Autodesk Fusion 360 part; units mm, degrees
note: some values were not read from the file. Set by a fixed rule: which face or edge a step refers to.
(part 4 of 4)
sketch "Sketch2 (2)" plane through (0, 0, 5) normal (0, 0, 1) x (-1, 0, 0)
  line L0 (3.02, 3.0627) -> (-2.5, 1.0536)
  line L1 (-2.5, 1.0536) -> (-2.5, -1.0536)
  line L2 (-2.5, -1.0536) -> (3.02, -3.0627)
  line L3 (3.02, -3.0627) -> (3.02, -4.7913)
  line L4 (3.02, -4.7913) -> (-2.5, -6.8004)
  line L5 (-2.5, -6.8004) -> (-2.5, -8.9076)
  line L6 (-2.5, -8.9076) -> (3.02, -10.9167)
  line L7 (3.02, -10.9167) -> (3.02, -12.6453)
  line L8 (3.02, -12.6453) -> (-2.5, -14.6544)
  line L9 (-2.5, -14.6544) -> (-2.5, -16.7615)
  line L10 (-2.5, -16.7615) -> (3.02, -18.7706)
  line L11 (3.02, -18.7706) -> (3.02, -20.4993)
  line L12 (3.02, -20.4993) -> (-2.5, -22.5084)
  line L13 (-2.5, -22.5084) -> (-2.5, -24.6155)
  line L14 (-2.5, -24.6155) -> (3.02, -26.6246)
  line L15 (3.02, -26.6246) -> (3.02, -28.3532)
  line L16 (3.02, -28.3532) -> (-2.5, -30.3624)
  line L17 (-2.5, -30.3624) -> (-2.5, -32.4695)
  line L18 (-2.5, -32.4695) -> (3.02, -34.4786)
  line L19 (3.02, -34.4786) -> (3.02, -36.2072)
  line L20 (3.02, -36.2072) -> (-2.5, -38.2163)
  line L21 (-2.5, -38.2163) -> (-2.5, -40.3235)
  line L22 (-2.5, -40.3235) -> (3.02, -42.3326)
  line L23 (3.02, -42.3326) -> (3.02, -44.0612)
  line L24 (3.02, -44.0612) -> (-2.5, -46.0703)
  line L25 (-2.5, -46.0703) -> (-2.5, -48.1775)
  line L26 (-2.5, -48.1775) -> (3.02, -50.1866)
  line L27 (3.02, -50.1866) -> (3.02, -51.9152)
  line L28 (3.02, -51.9152) -> (-2.5, -53.9243)
  line L29 (-2.5, -53.9243) -> (-2.5, -56.0314)
  line L30 (-2.5, -56.0314) -> (3.02, -58.0406)
  line L31 (3.02, -58.0406) -> (3.02, -59.7692)
  line L32 (3.02, -59.7692) -> (-2.5, -61.7783)
  line L33 (-2.5, -61.7783) -> (-2.5, -63.8854)
  line L34 (-2.5, -63.8854) -> (3.02, -65.8945)
  line L35 (3.02, -65.8945) -> (3.02, -67.6231)
  line L36 (3.02, -67.6231) -> (-2.5, -69.6323)
  line L37 (-2.5, -69.6323) -> (-2.5, -71.7394)
  line L38 (-2.5, -71.7394) -> (3.02, -73.7485)
  line L39 (3.02, -73.7485) -> (3.02, -75.4771)
  line L40 (3.02, -75.4771) -> (-2.5, -77.4862)
  line L41 (-2.5, -77.4862) -> (-2.5, -79.5934)
  line L42 (-2.5, -79.5934) -> (3.02, -81.6025)
  line L43 (3.02, -81.6025) -> (3.02, -83.3311)
  line L44 (3.02, -83.3311) -> (-2.5, -85.3402)
  line L45 (-2.5, -85.3402) -> (-2.5, -87.4474)
  line L46 (-2.5, -87.4474) -> (3.02, -89.4565)
  line L47 (3.02, -89.4565) -> (3.02, -91.1851)
  line L48 (3.02, -91.1851) -> (-2.5, -93.1942)
  line L49 (-2.5, -93.1942) -> (-2.5, -95.3013)
  line L50 (-2.5, -95.3013) -> (3.02, -97.3105)
  line L51 (3.02, -97.3105) -> (3.02, -99.0391)
  line L52 (3.02, -99.0391) -> (-2.5, -101.0482)
  line L53 (-2.5, -101.0482) -> (-2.5, -103.1553)
  line L54 (-2.5, -103.1553) -> (3.02, -105.1644)
  line L55 (3.02, -105.1644) -> (3.02, -106.8931)
  line L56 (3.02, -106.8931) -> (-2.5, -108.9022)
  line L57 (-2.5, -108.9022) -> (-2.5, -111.0093)
  line L58 (-2.5, -111.0093) -> (3.02, -113.0184)
  line L59 (3.02, -113.0184) -> (3.02, -114.747)
  line L60 (3.02, -114.747) -> (-2.5, -116.7562)
  line L61 (-2.5, -116.7562) -> (-2.5, -118.8633)
  line L62 (-2.5, -118.8633) -> (3.02, -120.8724)
  line L63 (3.02, -120.8724) -> (3.02, -122.601)
  line L64 (3.02, -122.601) -> (-2.5, -124.6101)
  line L65 (-2.5, -124.6101) -> (-2.5, -126.7173)
  line L66 (-2.5, -126.7173) -> (3.02, -128.7264)
  line L67 (3.02, -128.7264) -> (3.02, -130.455)
  line L68 (3.02, -130.455) -> (-2.5, -132.4641)
  line L69 (-2.5, -132.4641) -> (-2.5, -134.5713)
  line L70 (-2.5, -134.5713) -> (3.02, -136.5804)
  line L71 (3.02, -136.5804) -> (3.02, -138.309)
  line L72 (3.02, -138.309) -> (-2.5, -140.3181)
  line L73 (-2.5, -140.3181) -> (-2.5, -142.4252)
  line L74 (-2.5, -142.4252) -> (3.02, -144.4344)
  line L75 (3.02, -144.4344) -> (3.02, -146.163)
  line L76 (3.02, -146.163) -> (-2.5, -148.1721)
  line L77 (-2.5, -148.1721) -> (-2.5, -150.2792)
  line L78 (-2.5, -150.2792) -> (3.02, -152.2883)
  line L79 (3.02, -152.2883) -> (3.02, -154.0169)
  line L80 (3.02, -154.0169) -> (-2.5, -156.0261)
  line L81 (-2.5, -156.0261) -> (-2.5, -158.1332)
  line L82 (-2.5, -158.1332) -> (3.02, -160.1423)
  line L83 (3.02, -160.1423) -> (3.02, -161.8709)
  line L84 (3.02, -161.8709) -> (-2.5, -163.88)
  line L85 (-2.5, -163.88) -> (-2.5, -165.9872)
  line L86 (-2.5, -165.9872) -> (3.02, -167.9963)
  line L87 (3.02, -167.9963) -> (3.02, -169.7249)
  line L88 (3.02, -169.7249) -> (-2.5, -171.734)
  line L89 (-2.5, -171.734) -> (-2.5, -173.8412)
  line L90 (-2.5, -173.8412) -> (3.02, -175.8503)
  line L91 (3.02, -175.8503) -> (3.02, -177.5789)
  line L92 (3.02, -177.5789) -> (-2.5, -179.588)
  line L93 (-2.5, -179.588) -> (-2.5, -181.6951)
  line L94 (-2.5, -181.6951) -> (3.02, -183.7043)
  line L95 (3.02, -183.7043) -> (3.02, -184.5686)
  line L96 (3.02, -184.5686) -> (13.02, -184.5686)
  line L97 (13.02, -184.5686) -> (13.02, 18.927)
  line L98 (13.02, 18.927) -> (-76.98, 18.927)
  line L99 (-76.98, 18.927) -> (-76.98, 3.927)
  line L100 (-76.98, 3.927) -> (3.02, 3.927)
  line L101 (3.02, 3.927) -> (3.02, 3.0627)
  line L102 (-31.98, 18.927) -> (-31.98, 3.927) construction
  line L103 (-76.98, 3.927) -> (-31.98, 18.927) construction
  line L104 (13.02, 3.927) -> (-31.98, 18.927) construction
  line L105 (-36.98, 15.177) -> (-26.98, 15.177)
  line L106 (-26.98, 15.177) -> (-26.98, 7.677)
  line L107 (-26.98, 7.677) -> (-36.98, 7.677)
  line L108 (-36.98, 7.677) -> (-36.98, 15.177)
  line L109 (-36.98, 15.177) -> (-26.98, 7.677) construction
  line L110 (-26.98, 15.177) -> (-36.98, 7.677) construction
  line L111 (-14.48, 15.177) -> (-4.48, 15.177)
  line L112 (-4.48, 15.177) -> (-4.48, 7.677)
  line L113 (-4.48, 7.677) -> (-14.48, 7.677)
  line L114 (-14.48, 7.677) -> (-14.48, 15.177)
  line L115 (-14.48, 15.177) -> (-4.48, 7.677) construction
  line L116 (-4.48, 15.177) -> (-14.48, 7.677) construction
  point P0 (-31.98, 11.427)
  point P1 (-54.48, 11.427)
  point P2 (-9.48, 11.427)
  dimension "d8" = 10
  dimension "d9" = 7.5
  dimension "d12" = 10
  dimension "d13" = 7.5
  constraint midpoint L98 L102.start
  constraint coincident L100 L102.end
  constraint perpendicular L100 L102
  constraint coincident L99.end L100.start
  constraint coincident L97 L104.start
  constraint horizontal L105
  constraint perpendicular L105 L106
  constraint parallel L105 L107
  constraint parallel L106 L108
  constraint coincident L109 P0
  constraint coincident L110 P0
  constraint midpoint L102 P0
  constraint midpoint L103 P1
  constraint horizontal L111
  constraint perpendicular L111 L112
  constraint parallel L111 L113
  constraint parallel L112 L114
  constraint coincident L115 P2
  constraint coincident L116 P2
  constraint midpoint L104 P2
  measures "d8" distance of L105.start L105.end
  measures "d9" distance of L105.start L107.end
  measures "d12" distance of L111.start L111.end
  measures "d13" distance of L111.end L112.end
extrude "Extrude3" cut sketch "Sketch2 (2)" against normal blind 10 contours L105 L106 L107 L108 | L111 L112 L113 L114 in component "Rack; Module: 2.50 mm; Num Teeth: 24; Pressure Angle: 20 deg; Backlash: 0.00 mm;"
sketch "Sketch3" plane through (0, -18.927, 0) normal (0, -1, 0) x (1, 0, 0)
  line L0 (76.98, 5) -> (-13.02, 5)
  line L1 (-13.02, 5) -> (-13.02, -5)
  line L2 (-13.02, -5) -> (76.98, -5)
  line L3 (76.98, -5) -> (76.98, 5)
  line L4 (31.98, 5) -> (31.98, -5) construction
  line L5 (-13.02, 5) -> (31.98, -5) construction
  line L6 (76.98, 5) -> (31.98, -5) construction
  circle A0 centre (31.98, 0) radius 1.5
  circle A1 centre (9.48, 0) radius 1.5
  dimension "d16" = 3
  dimension "d17" = 3
  constraint midpoint L0 L4.start
  constraint midpoint L2 L4.end
  constraint coincident L0.end L1.start
  constraint coincident L0.start L3.end
  constraint midpoint L4 A0.centre
  constraint midpoint L5 A1.centre
  measures "d16" diameter of A1
  measures "d17" diameter of A0
extrude "Extrude4" cut sketch "Sketch3" against normal blind 15 contours A0 | A1 in component "Rack; Module: 2.50 mm; Num Teeth: 24; Pressure Angle: 20 deg; Backlash: 0.00 mm;"
extrude "Extrude5" cut 1 faces at (76.98, -8.927, -1.6667) along direction (-1, 0, 0) blind 20 in component "Rack; Module: 2.50 mm; Num Teeth: 24; Pressure Angle: 20 deg; Backlash: 0.00 mm;"
sketch "Sketch4" plane through (0, 184.5686, 0) normal (0, 1, 0) x (-1, 0, 0)
  line L0 (13.02, -5) -> (13.02, 5)
  line L1 (13.02, 5) -> (3.02, 5)
  line L2 (3.02, 5) -> (3.02, -5)
  line L3 (3.02, -5) -> (13.02, -5)
  line L4 (13.02, 5) -> (-13, 5)
  line L5 (-13, 5) -> (-13, -5)
  line L6 (-13, -5) -> (13.02, -5)
  line L7 (13.02, -5) -> (13.02, 5)
  constraint perpendicular L4 L5
  constraint parallel L4 L6
  constraint parallel L5 L7
  constraint perpendicular L0 L4
  constraint coincident L0.end L1.start
extrude "Extrude6" cut sketch "Sketch4" against normal blind 31 in component "Rack; Module: 2.50 mm; Num Teeth: 24; Pressure Angle: 20 deg; Backlash: 0.00 mm;"
component "Rack; Module: 2.50 mm; Num Teeth: 24; Pressure Angle: 20 deg; Backlash: 0.00 mm;" placed x (1, 0, 0) y (0, 1, 0) z (0, 0, 1) at (0, 0, 0)

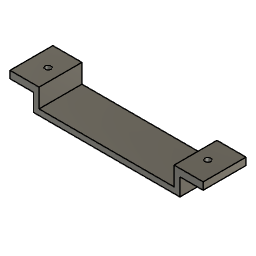
design "bracket"
Autodesk Fusion 360 part; units mm, degrees
sketch "Sketch1" plane through (0, 0, 0) normal (0, 0, 1) x (1, 0, 0)
  line L0 (50.5, -44.75) -> (-50.5, -44.75)
  line L1 (-50.5, -44.75) -> (-50.5, 44.75)
  line L2 (-50.5, 44.75) -> (50.5, 44.75)
  line L3 (50.5, 44.75) -> (50.5, -44.75)
  line L4 (50.5, -44.75) -> (-50.5, 44.75) construction
  line L5 (-50.5, -44.75) -> (50.5, 44.75) construction
  dimension "d1" = 101
  dimension "d2" = 89.5
  constraint horizontal L0
  constraint perpendicular L0 L1
  constraint parallel L0 L2
  constraint parallel L1 L3
  constraint coincident L4 origin
  constraint coincident L5 origin
  measures "d1" distance of L1.end L2.end
  measures "d2" distance of L0.end L1.end
extrude "Extrude1" add sketch "Sketch1" along normal blind 12
shell "Shell1" thickness 4 removed faces 1 at (-16.8333, 14.9167, 12)
extrude "Extrude2" cut 1 faces at (15.5, 40.75, 6.6667) along direction (0, -1, 0) up to surface (85.5 mm away) and the other way up to surface (4 mm away)
sketch "Sketch3" plane through (0, 0, 12) normal (0, 0, 1) x (-1, 0, 0)
  line L0 (46.5, 44.75) -> (46.5, -44.75)
  line L1 (46.5, -44.75) -> (50.5, -44.75)
  line L2 (50.5, -44.75) -> (50.5, 44.75)
  line L3 (50.5, 44.75) -> (46.5, 44.75)
  line L4 (46.5, -44.75) -> (66.5, -44.75)
  line L5 (66.5, -44.75) -> (66.5, 44.75)
  line L6 (66.5, 44.75) -> (46.5, 44.75)
  line L7 (46.5, 44.75) -> (46.5, -44.75)
  line L8 (0, -2.5) -> (0, -20)
  line L9 (-46.5, -44.75) -> (-66.5, -44.75)
  line L10 (-66.5, -44.75) -> (-66.5, 44.75)
  line L11 (-46.5, 44.75) -> (-46.5, -44.75)
  line L12 (-66.5, 44.75) -> (-46.5, 44.75)
  line L13 (0, 0) -> (55, 0) construction
  circle A0 centre (55, 0) radius 2
  circle A1 centre (-55, 0) radius 2
  dimension "d15" = 89.5
  dimension "d16" = 20
  dimension "d21" = 55
  dimension "d22" = 4
  constraint perpendicular L4 L5
  constraint parallel L4 L6
  constraint parallel L5 L7
  constraint perpendicular L2 L4
  constraint coincident L0.end L1.start
  constraint symmetric L0.end L8 L9.start
  constraint symmetric L4.end L8 L9.end
  constraint symmetric L5.end L8 L10.end
  constraint symmetric L0.start L8 L11.start
  constraint coincident L13.start origin
  constraint perpendicular L2 L13
  constraint coincident L13.end A0.centre
  constraint symmetric L8 A0 A1
  measures "d15" distance of L4.end L5.end
  measures "d16" distance of L5.end L0.start
  measures "d21" distance of L13.start L13.end
  measures "d22" diameter of A0
extrude "Extrude4" add sketch "Sketch3" along normal blind 5
move_face "OffsetFaces1" offset -30 1 faces at (54.5, -44.75, 15.3333)
move_face "OffsetFaces2" offset -30 1 faces at (54.5, 44.75, 15.3333)

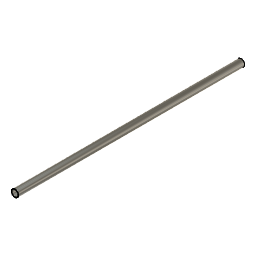
design "axle"
Autodesk Fusion 360 part; units mm, degrees
sketch "Sketch1" plane through (0, 0, 0) normal (0, 1, 0) x (1, 0, 0)
  circle A0 centre (0, 0) radius 4
  circle A1 centre (0, 0) radius 3.5
  dimension "d1" = 8
  dimension "d2" = 7
  constraint coincident A0.centre A1.centre
  measures "d1" diameter of A0
  measures "d2" diameter of A1
extrude "Extrude1" add sketch "Sketch1" along normal mid plane 250

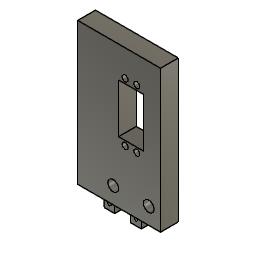
design "servo_side_stand"
Autodesk Fusion 360 part; units mm, degrees
sketch "Sketch1" plane through (0, 0, 0) normal (0, 0, 1) x (1, 0, 0)
  line L0 (45, -7.5) -> (-45, -7.5) construction
  line L1 (-45, -7.5) -> (-45, 7.5) construction
  line L2 (-45, 7.5) -> (45, 7.5) construction
  line L3 (45, 7.5) -> (45, -7.5) construction
  line L4 (45, -7.5) -> (-45, 7.5) construction
  line L5 (-45, -7.5) -> (45, 7.5) construction
  line L6 (0, -7.5) -> (45, 7.5) construction
  line L7 (-45, 7.5) -> (0, -7.5) construction
  line L8 (4.5, -3.25) -> (-4.5, -3.25)
  line L9 (-4.5, -3.25) -> (-4.5, 3.25)
  line L10 (-4.5, 3.25) -> (4.5, 3.25)
  line L11 (4.5, 3.25) -> (4.5, -3.25)
  line L12 (4.5, -3.25) -> (-4.5, 3.25) construction
  line L13 (-4.5, -3.25) -> (4.5, 3.25) construction
  line L14 (-27, -3.25) -> (-18, -3.25)
  line L15 (-18, -3.25) -> (-18, 3.25)
  line L16 (-18, 3.25) -> (-27, 3.25)
  line L17 (-27, 3.25) -> (-27, -3.25)
  line L18 (-27, -3.25) -> (-18, 3.25) construction
  line L19 (-18, -3.25) -> (-27, 3.25) construction
  point P0 (22.5, 0)
  point P1 (-22.5, 0)
  dimension "d1" = 90
  dimension "d2" = 15
  dimension "d3" = 9
  dimension "d4" = 9
  dimension "d7" = 6.5
  dimension "d8" = 6.5
  constraint horizontal L0
  constraint perpendicular L0 L1
  constraint parallel L0 L2
  constraint parallel L1 L3
  constraint coincident L4 origin
  constraint coincident L5 origin
  constraint midpoint L0 L6.start
  constraint horizontal L8
  constraint perpendicular L8 L9
  constraint parallel L8 L10
  constraint parallel L9 L11
  constraint coincident L12 origin
  constraint coincident L13 origin
  constraint midpoint L6 P0
  constraint horizontal L14
  constraint perpendicular L14 L15
  constraint parallel L14 L16
  constraint parallel L15 L17
  constraint coincident L18 P1
  constraint coincident L19 P1
  constraint midpoint L7 P1
  measures "d1" distance of L0.start L0.end
  measures "d2" distance of L0.end L1.end
  measures "d3" distance of L14.start L14.end
  measures "d4" distance of L8.start L8.end
  measures "d7" distance of L8.start L10.end
  measures "d8" distance of L14.end L15.end
extrude "Extrude1" add sketch "Sketch1" along normal blind 10 makes body 1 at (-21, 3.25, 3.3333) makes body 2 at (-1.5, 3.25, 3.3333)
sketch "Sketch2" plane through (0, 0, 10) normal (0, 0, 1) x (-1, 0, 0)
  line L0 (45, 7.5) -> (-45, 7.5)
  line L1 (-45, 7.5) -> (-45, -7.5)
  line L2 (-45, -7.5) -> (45, -7.5)
  line L3 (45, -7.5) -> (45, 7.5)
  line L4 (45, 7.5) -> (-45, -7.5) construction
  line L5 (-45, 7.5) -> (45, -7.5) construction
  line L6 (27, -3.25) -> (27, 3.25)
  line L7 (27, 3.25) -> (18, 3.25)
  line L8 (18, 3.25) -> (18, -3.25)
  line L9 (18, -3.25) -> (27, -3.25)
  line L10 (-4.5, -3.25) -> (4.5, -3.25)
  line L11 (4.5, -3.25) -> (4.5, 3.25)
  line L12 (4.5, 3.25) -> (-4.5, 3.25)
  line L13 (-4.5, 3.25) -> (-4.5, -3.25)
  dimension "d11" = 90
  dimension "d12" = 15
  constraint horizontal L0
  constraint perpendicular L0 L1
  constraint parallel L0 L2
  constraint parallel L1 L3
  constraint coincident L4 origin
  constraint coincident L5 origin
  measures "d11" distance of L0.start L0.end
  measures "d12" distance of L0.start L2.end
extrude "Extrude2" add sketch "Sketch2" along normal blind 120 contours L0 L1 L2 L3 | L6 L7 L8 L9 | L10 L11 L12 L13 bodies 1 2
sketch "Sketch3" plane through (0, -7.5, 0) normal (0, -1, 0) x (1, 0, 0)
  line L0 (-45, 10) -> (45, 10)
  line L1 (45, 10) -> (45, 130)
  line L2 (45, 130) -> (-45, 130)
  line L3 (-45, 130) -> (-45, 10)
  line L4 (0, 10) -> (0, 82.9) construction
  line L5 (10.5, 62.15) -> (-10.5, 62.15)
  line L6 (-10.5, 62.15) -> (-10.5, 103.65)
  line L7 (-10.5, 103.65) -> (10.5, 103.65)
  line L8 (10.5, 103.65) -> (10.5, 62.15)
  line L9 (10.5, 62.15) -> (-10.5, 103.65) construction
  line L10 (-10.5, 62.15) -> (10.5, 103.65) construction
  line L11 (10, 58.15) -> (-10, 58.15) construction
  line L12 (-10, 58.15) -> (-10, 107.65) construction
  line L13 (-10, 107.65) -> (10, 107.65) construction
  line L14 (10, 107.65) -> (10, 58.15) construction
  line L15 (10, 58.15) -> (-10, 107.65) construction
  line L16 (-10, 58.15) -> (10, 107.65) construction
  circle A0 centre (4.925, 107.65) radius 2.5
  line L17 (0, 107.65) -> (0, 82.9) construction
  circle A1 centre (-4.925, 107.65) radius 2.5
  line L18 (0, 82.9) -> (10, 82.9) construction
  circle A2 centre (-4.925, 58.15) radius 2.5
  circle A3 centre (4.925, 58.15) radius 2.5
  point P0 (0, 82.9)
  point P1 (0, 82.9)
  point P2 (4.925, 107.65)
  dimension "d15" = 72.9
  dimension "d16" = 41.5
  dimension "d17" = 21
  dimension "d18" = 20
  dimension "d19" = 49.5
  dimension "d20" = 4.925
  dimension "d21" = 5
  constraint midpoint L0 L4.start
  constraint perpendicular L0 L4
  constraint horizontal L5
  constraint perpendicular L5 L6
  constraint parallel L5 L7
  constraint parallel L6 L8
  constraint coincident L9 P1
  constraint coincident L10 P1
  constraint coincident P1 P0
  constraint horizontal L11
  constraint perpendicular L11 L12
  constraint parallel L11 L13
  constraint parallel L12 L14
  constraint coincident L15 P1
  constraint coincident L16 P1
  constraint coincident L13 P2
  constraint coincident P2 A0.centre
  constraint symmetric A0 L17 A1
  constraint midpoint L14 L18.end
  constraint symmetric A0 L18 A3
  constraint symmetric A1 L18 A2
  measures "d15" distance of L4.start P1
  measures "d16" distance of L5.end L6.end
  measures "d17" distance of L6.end L7.end
  measures "d18" distance of L12.end L13.end
  measures "d19" distance of L11.start L13.end
  measures "d20" distance of P2 L17.start
  measures "d21" diameter of A0
extrude "Extrude3" cut sketch "Sketch3" against normal blind 15 contours L5 L6 L7 L8 | A0 | A1 | A2 | A3 bodies 1
sketch "Sketch4" plane through (0, -3.25, 0) normal (0, -1, 0) x (1, 0, 0)
  line L0 (-27, 0) -> (-18, 0)
  line L1 (-18, 0) -> (-18, 10)
  line L2 (-18, 10) -> (-27, 10)
  line L3 (-27, 10) -> (-27, 0)
  line L4 (-27, 10) -> (-18, 0) construction
  circle A0 centre (-22.5, 5) radius 1.5
  line L5 (-4.5, 10) -> (4.5, 0)
  circle A1 centre (0, 5) radius 1.5
  dimension "d24" = 3
  dimension "d41" = 22.5
  dimension "d42" = 0
  constraint coincident L2.end L3.start
  constraint coincident L0.end L1.start
  constraint midpoint L4 A0.centre
  measures "d24" diameter of A0
extrude "Extrude4" cut sketch "Sketch4" against normal blind 10 contours A0 | L5 A1 | L5 A1 bodies 1
extrude "Extrude5" cut 1 faces at (45, -2.5, 50) along direction (-1, 0, 0) blind 20 on bodies 1 bodies 1
sketch "Sketch5" plane through (0, -7.5, 0) normal (0, -1, 0) x (1, 0, 0)
  line L0 (25, 10) -> (25, 130)
  line L1 (25, 130) -> (-45, 130)
  line L2 (-45, 130) -> (-45, 10)
  line L3 (-45, 10) -> (25, 10)
  circle A0 centre (4.925, 107.65) radius 2.5
  circle A1 centre (-4.925, 107.65) radius 2.5
  circle A2 centre (-4.925, 58.15) radius 2.5
  line L4 (-10.5, 62.15) -> (-10.5, 103.65)
  line L5 (-10.5, 103.65) -> (10.5, 103.65)
  line L6 (10.5, 103.65) -> (10.5, 62.15)
  line L7 (10.5, 62.15) -> (-10.5, 62.15)
  circle A3 centre (4.925, 58.15) radius 2.5
  line L8 (0, 10) -> (15, 10) construction
  line L9 (0, 10) -> (-15, 10) construction
  line L10 (-15, 10) -> (-15, 24) construction
  line L11 (15, 10) -> (15, 24) construction
  circle A4 centre (-15, 24) radius 4.5
  circle A5 centre (15, 24) radius 4.5
  dimension "d31" = 15
  dimension "d32" = 15
  dimension "d33" = 9
  dimension "d34" = 9
  dimension "d37" = 14
  dimension "d38" = 14
  constraint horizontal L8
  constraint parallel L3 L9
  constraint perpendicular L3 L10
  constraint perpendicular L3 L11
  constraint coincident L10.end A4.centre
  constraint coincident L11.end A5.centre
  measures "d31" distance of L8.start L9.end
  measures "d32" distance of L8.start L8.end
  measures "d33" diameter of A4
  measures "d34" diameter of A5
  measures "d37" distance of L9.end L10.end
  measures "d38" distance of L8.end L11.end
extrude "Extrude6" cut sketch "Sketch5" against normal up to surface (15 mm away) contours A4 | A5 bodies 1
